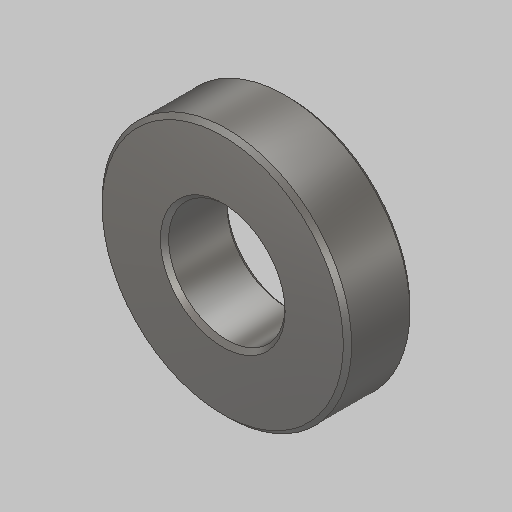
# Autodesk Inventor part: 0_875_ID_x_1_875_OD_X_0_500_Radial_Bearing_EE11S-2RS
Saved by Autodesk Inventor 2023.5 (Build 275446000, 446)
## iProperties
Created: 2023-01-21
Part Number: 0_875_ID_x_1_875_OD_X_0_500_Radial_Bearing_EE11S-2RS
Material: Steel, Mild
Document SubType Name: Modeling
Designer: mavericks
Density: 7.85 g/cm^3
Appearance: Semi-Polished
Mass: 137.838 g
Surface Area: 53.7004 cm^2
Volume: 17.5589 cm^3
Author: mavericks
Autodesk Inventor part; units mm, degrees
ref_plane "YZ Plane" through (0, 0, 0) normal (1, 0, 0) x (0, 1, 0)
ref_plane "XZ Plane" through (0, 0, 0) normal (0, 1, 0) x (-1, 0, 0)
ref_plane "XY Plane" through (0, 0, 0) normal (0, 0, 1) x (1, 0, 0)
sketch "Sketch1" plane through (0, 0, 0) normal (0, 0, 1) x (1, 0, 0)
  circle A0 centre (0, 0) radius 23.8125
  circle A1 centre (0, 0) radius 11.1125
  dimension "d0" = 47.625
  dimension "d1" = 22.225
  constraints: 2 centre point, 2 coincident
  measures "d0" diameter of A0
  measures "d1" diameter of A1
extrude "Extrusion1" add sketch "Sketch1" along normal blind 12.7
chamfer "Chamfer1" distance 0.7925 angle 45 4 edges at (-11.1125, 0, 12.7) (-11.1125, 0, 0) (-23.8125, 0, 12.7) (-23.8125, 0, 0)
body "Solid1"
